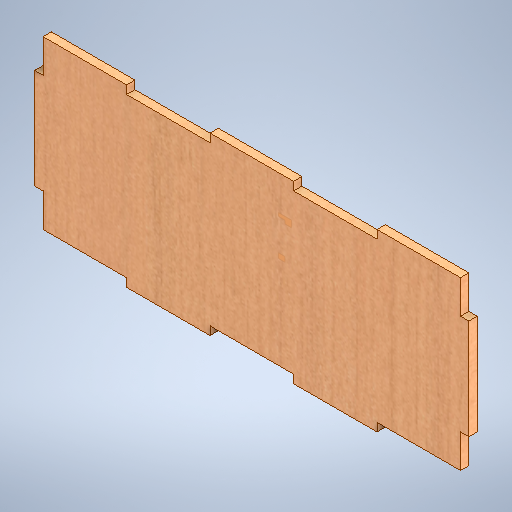
# Autodesk Inventor part: Lat1(2)
Saved by Autodesk Inventor 2025 (Build 290162000, 162)
## iProperties
Created: 2024-11-02
Part Number: Lat1(2)
Material: Wood (Cherry)
Document SubType Name: Sheet Metal
Designer: g.marin
Density: 0.63 g/cm^3
Sheet Metal Rule: Default
Appearance: Cherry - Natural Low Gloss
Author: g.marin
Autodesk Inventor part; units mm, degrees
ref_plane "YZ Plane" through (0, 0, 0) normal (1, 0, 0) x (0, 1, 0)
ref_plane "XZ Plane" through (0, 0, 0) normal (0, 1, 0) x (-1, 0, 0)
ref_plane "XY Plane" through (0, 0, 0) normal (0, 0, 1) x (1, 0, 0)
sketch "Sketch1" plane through (0, 0, 0) normal (0, 0, 1) x (1, 0, 0)
  line L0 (-130, -50) -> (130, -50)
  line L1 (130, -50) -> (130, 50)
  line L2 (130, 50) -> (-130, 50)
  line L3 (-130, 50) -> (-130, -50)
  line L4 (-130, -50) -> (130, 50) construction
  line L5 (130, -50) -> (-130, 50) construction
  line L6 (-75, -50) -> (-25, -50)
  line L7 (-25, -50) -> (-25, -55)
  line L8 (-25, -55) -> (-75, -55)
  line L9 (-75, -55) -> (-75, -50)
  line L10 (25, -50) -> (75, -50)
  line L11 (75, -50) -> (75, -55)
  line L12 (75, -55) -> (25, -55)
  line L13 (25, -55) -> (25, -50)
  line L14 (130, 50) -> (125, 50)
  line L15 (125, 50) -> (125, 30)
  line L16 (125, 30) -> (130, 30)
  line L17 (130, 30) -> (130, 50)
  line L18 (130, -50) -> (125, -50)
  line L19 (125, -50) -> (125, -30)
  line L20 (125, -30) -> (130, -30)
  line L21 (130, -30) -> (130, -50)
  line L22 (0, 50) -> (0, -50) construction
  line L23 (-125, 50) -> (-125, 30)
  line L24 (-125, 30) -> (-130, 30)
  line L25 (-125, -50) -> (-125, -30)
  line L26 (-125, -30) -> (-130, -30)
  line L27 (-75, 50) -> (-25, 50)
  line L28 (-25, 50) -> (-25, 45)
  line L29 (-25, 45) -> (-75, 45)
  line L30 (-75, 45) -> (-75, 50)
  line L31 (25, 50) -> (75, 50)
  line L32 (75, 50) -> (75, 45)
  line L33 (75, 45) -> (25, 45)
  line L34 (25, 45) -> (25, 50)
  point P0 (0, 0)
  point P1 (-75, -52.5)
  point P2 (-25, -50)
  point P3 (75, -50)
  point P4 (-125, -50)
  point P5 (130, -30)
  point P6 (130, 30)
  point P7 (125, 50)
  point P8 (-125, 50)
  point P9 (-130, 30)
  point P10 (75, 50)
  point P11 (-25, 50)
  dimension "d0" = 260
  dimension "d1" = 100
  dimension "d2" = 50
  dimension "d3" = 50
  dimension "d4" = 50
  dimension "d5" = 55
  dimension "d6" = 5
  dimension "d10" = 20
  dimension "d12" = 5
  dimension "d13" = 50
  dimension "d14" = 50
  dimension "d15" = 5
  dimension "d16" = 20
  constraints: 70 end point, 14 parallel, 8 point on line, 7 horizontal, 7 perpendicular, 6 symmetric about line, 5 midpoint, 2 collinear
  measures "d0" distance of L1.end L2.end
  measures "d1" distance of L0.end L1.end
  measures "d2" distance of L7.end L8.end
  measures "d3" distance of L11.end L12.end
  measures "d4" distance between parallel lines of L13 L7
  measures "d5" horizontal distance of point (-75, -52.5) L0.start
  measures "d6" distance of L6.end L7.end
  measures "d10" distance of L18.end L19.end
  measures "d12" distance of L15.end L16.end
  measures "d13" distance of L28.end L29.end
  measures "d14" distance of L32.end L33.end
  measures "d15" distance of L29.end L27.start
  measures "d16" distance of L14.end L15.end
extrude "Extrusion1" add sketch "Sketch1" along normal blind 5 contours L25 L26 L3 L24 L23 L2 L30 L29 L28 L34 L33 L32 L15 L16 L1 L20 L19 L0 | L0 L7 L8 L9 | L0 L11 L12 L13
equation "\"BendRadius\" = Thickness"
equation "\"BendReliefWidth\" = Thickness"
equation "\"BendReliefDepth\" = 0.5 * Thickness"
equation "\"CornerReliefSize\" = 4 * Thickness"
equation "\"MinimumRemnant\" = 2 * Thickness"
equation "\"TransitionRadius\" = BendRadius"
equation "\"JacobiRadiusSize\" = BendRadius"
equation "\"GapSize\" = Thickness"
equation "\"Thickness\" = 3.048"
body "Solid1"
